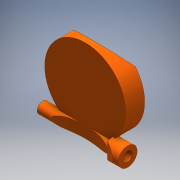
# Autodesk Inventor part: Loquet Haut
Saved by Autodesk Inventor 2016 SP1 (Build 200210100, 210)
## iProperties
Created: 2017-04-27
Part Number: Loquet Haut
Material: Plastique ABS
Document SubType Name: Modeling
Designer: dimercur
Density: 1.06 g/cm^3
Appearance: Lisse - Orange clair
Author: dimercur
Autodesk Inventor part; units mm, degrees
ref_plane "YZ Plane" through (0, 0, 0) normal (1, 0, 0) x (0, 1, 0)
ref_plane "XZ Plane" through (0, 0, 0) normal (0, 1, 0) x (-1, 0, 0)
sketch "Esquisse1" plane through (0, 0, 0) normal (0, 1, 0) x (-1, 0, 0)
  circle A0 centre (0, 0) radius 21.5
  dimension "d0" = 43
  constraints: 1 centre point, 1 coincident
  measures "d0" diameter of A0
extrude "Extrusion1" add sketch "Esquisse1" along normal mid plane 40
sketch "Esquisse2" plane through (0, 0, 0) normal (0, 0, 1) x (1, 0, 0)
  circle A0 centre (0, 25) radius 23
  line L0 (-28, -1) -> (28, -1)
  line L1 (28, -1) -> (28, -20)
  line L2 (28, -20) -> (-28, -20)
  line L3 (-28, -20) -> (-28, -1)
  point P0 (0, 0)
  dimension "d3" = 25
  dimension "d4" = 46
  dimension "d8" = 1
  dimension "d9" = 56
  dimension "d10" = 28
  dimension "d11" = 19
  constraints: 8 end point, 2 parallel, 1 centre point, 1 horizontal, 1 perpendicular
  measures "d3" distance of point (0, 0) A0.centre
  measures "d4" diameter of A0
  measures "d8" distance from line of point (0, 0) L0
  measures "d9" distance between parallel lines of L1 L3
  measures "d10" distance from line of point (0, 0) L3
  measures "d11" distance of L2.end L0.start
extrude "Extrusion2" cut sketch "Esquisse2" along normal through all both and the other way through all
sketch "Esquisse13" plane through (0, -1, 0) normal (0, -1, 0) x (1, 0, 0)
  line L0 (-22.5, -22.5) -> (22.5, -22.5)
  line L1 (22.5, -22.5) -> (22.5, -16.5)
  line L2 (22.5, -16.5) -> (-22.5, -16.5)
  line L3 (-22.5, -16.5) -> (-22.5, -22.5)
  point P0 (0, 0)
  dimension "d56" = 6
  dimension "d57" = 45
  dimension "d58" = 22.5
  dimension "d59" = 16.5
  constraints: 8 end point, 2 parallel, 1 horizontal, 1 perpendicular
  measures "d56" distance of L0.end L1.end
  measures "d57" distance of L0.start L0.end
  measures "d58" distance from line of point (0, 0) L3
  measures "d59" vertical distance of point (0, 0) L1.end
extrude "Extrusion11" add sketch "Esquisse13" along normal mid plane 6
fillet "Congé7" radius 3 5 edges at (18.142, 2, -16.5) (0, 2, -22.5) (0, -4, -22.5) (0, -4, -16.5) (-18.142, 2, -16.5)
sketch "Esquisse17" plane through (22.5, -1, -19.5) normal (1, 0, 0) x (0, 0, -1)
  line L0 (-3, 0) -> (3, 0) projected
  circle A0 centre (0, 0) radius 5
  point P0 (-19.5, 1)
  dimension "d73" = 10
  constraints: 1 centre point, 1 midpoint
  measures "d73" diameter of A0
extrude "Extrusion14" add sketch "Esquisse17" against normal blind 8
sketch "Esquisse16" plane through (-22.5, -1, -19.5) normal (-1, 0, 0) x (0, 0, 1)
  line L0 (3, 0) -> (-3, 0) projected
  circle A0 centre (0, 0) radius 1.35
  point P0 (19.5, 1)
  dimension "d70" = 2.7
  constraints: 1 centre point, 1 midpoint
  measures "d70" diameter of A0
extrude "Extrusion13" cut sketch "Esquisse16" against normal blind 8
sketch "Esquisse18" plane through (22.5, -1, -19.5) normal (1, 0, 0) x (0, 0, -1)
  circle A0 centre (0, 0) radius 2.5
  point P0 (-19.5, 1)
  dimension "d76" = 5
  constraints: 1 centre point, 1 coincident
  measures "d76" diameter of A0
extrude "Extrusion15" cut sketch "Esquisse18" against normal blind 3.5
ref_plane "Plan de construction3" through (0, 0, 21.5) normal (0, 0, 1) x (1, 0, 0)
sketch "Esquisse19" plane through (0, 0, 21.5) normal (0, 0, 1) x (1, 0, 0)
  line L0 (-22.5, -4) -> (14.5, -4) projected
  circle A0 centre (0, -41) radius 40
  line L1 (21.5, -1) -> (-21.5, -1) projected
  point P0 (0, 0)
  point P1 (-13.784, -1)
  point P2 (15.8745, -1)
  dimension "d81" = 80
  dimension "d82" = 40
  constraints: 1 centre point
  measures "d81" diameter of A0
  measures "d82" distance from line of L1 A0.centre
extrude "Extrusion16" cut sketch "Esquisse19" against normal through all
sketch "Esquisse20" plane through (22.5, -1, -19.5) normal (1, 0, 0) x (0, 0, -1)
  line L0 (-35.0456, 22) -> (-0.0456, 22)
  line L1 (-0.0456, 22) -> (-0.0456, 10)
  line L2 (-0.0456, 10) -> (-35.0456, 10)
  line L3 (-35.0456, 10) -> (-35.0456, 22)
  line L4 (-3, 0) -> (-41, 0) projected
  point P0 (-19.5, 1)
  point P1 (-5, 0)
  dimension "d85" = 10
  dimension "d86" = 12
  dimension "d87" = 35
  constraints: 8 end point, 2 parallel, 1 horizontal, 1 perpendicular
  measures "d85" distance between parallel lines of L4 L2
  measures "d86" distance of L0.end L1.end
  measures "d87" distance of L0.start L0.end
extrude "Extrusion17" cut sketch "Esquisse20" against normal through all
equation "\"d10\" = 0.5 * d9"
equation "\"d82\" = 0.5 * d81"
